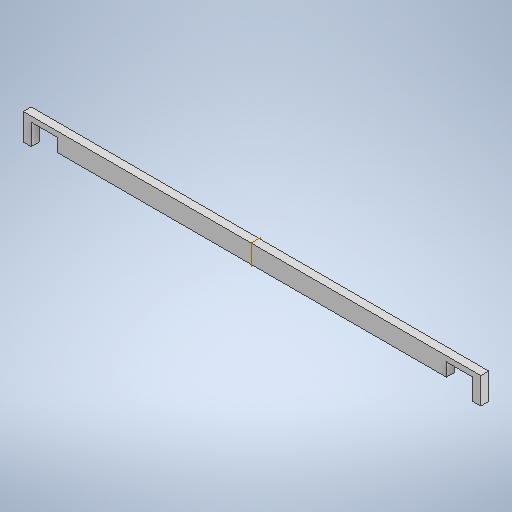
# Autodesk Inventor part: Bar
Saved by Autodesk Inventor 2025 (Build 290162010, 162A)
## iProperties
Created: 2024-06-06
Part Number: Bar
Material: Generic
Document SubType Name: Modeling
Designer: vncnt
Density: 1 g/cm^3
Appearance: Default
Author: vncnt
Autodesk Inventor part; units mm, degrees
ref_plane "YZ Plane" through (0, 0, 0) normal (1, 0, 0) x (0, 1, 0)
ref_plane "XZ Plane" through (0, 0, 0) normal (0, 1, 0) x (-1, 0, 0)
ref_plane "XY Plane" through (0, 0, 0) normal (0, 0, 1) x (1, 0, 0)
sketch "Sketch1" plane through (0, 0, 0) normal (0, 1, 0) x (-1, 0, 0)
  line L0 (-23.173, -32.8319) -> (-106.659, -32.8319)
  line L1 (-106.659, -32.8319) -> (-106.659, -34.3319)
  line L2 (-106.659, -34.3319) -> (-23.173, -34.3319)
  line L3 (-23.173, -34.3319) -> (-23.173, -32.8319)
  point P0 (0, 0)
  dimension "d0" = 83.486
  dimension "d1" = 1.5
  constraints: 8 end point, 2 parallel, 1 horizontal, 1 perpendicular
  measures "d0" distance of L1.end L2.end
  measures "d1" distance of L0.end L1.end
extrude "Extrusion1" add sketch "Sketch1" along normal blind 3.5
ref_plane "Work Plane1" through (64.916, 0, -32.8319) normal (1, 0, 0) x (0, 0, -1)
sketch "Sketch2" plane through (23.173, 0, -32.8319) normal (0, 0, 1) x (1, 0, 0)
  line L0 (83.486, 0) -> (78.486, 0)
  line L1 (78.486, 0) -> (78.486, 2.5)
  line L2 (78.486, 2.5) -> (83.486, 2.5)
  line L3 (83.486, 2.5) -> (83.486, 0)
  point P0 (-23.173, 0)
  dimension "d4" = 2.5
  dimension "d5" = 5
  constraints: 8 end point, 2 parallel, 1 horizontal, 1 perpendicular
  measures "d4" distance of L0.end L1.end
  measures "d5" distance of L1.end L2.end
extrude "Extrusion2" cut sketch "Sketch2" against normal blind 3.5
sketch "Sketch3" plane through (23.173, 3.5, -32.8319) normal (0, 0, 1) x (1, 0, 0)
  line L0 (0, 0) -> (83.486, 0) projected
  line L1 (83.486, 0) -> (84.986, 0)
  line L2 (84.986, 0) -> (84.986, -5)
  line L3 (84.986, -5) -> (83.486, -5)
  line L4 (83.486, -5) -> (83.486, 0)
  point P0 (-23.173, -3.5)
  dimension "d8" = 1.5
  dimension "d11" = 5
  constraints: 8 end point, 2 parallel, 1 horizontal, 1 perpendicular
  measures "d8" distance of L2.end L3.end
  measures "d11" distance of L1.end L2.end
extrude "Extrusion3" add sketch "Sketch3" against normal up to surface (1.5 mm away)
mirror "Mirror1" about plane through (64.916, 0, -32.8319) normal (1, 0, 0) of "Extrusion3", "Extrusion2"
body "Solid1"
